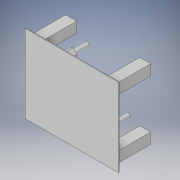
# Autodesk Inventor part: Protoboard
Saved by Autodesk Inventor 2019.3 (Build 233278000, 278)
## iProperties
Created: 2019-06-06
Part Number: Protoboard
Material: Generic
Document SubType Name: Modeling
Designer: Frienddo
Density: 1 g/cm^3
Appearance: Default
Author: Frienddo
Autodesk Inventor part; units mm, degrees
ref_plane "YZ Plane" through (0, 0, 0) normal (1, 0, 0) x (0, 1, 0)
ref_plane "XZ Plane" through (0, 0, 0) normal (0, 1, 0) x (-1, 0, 0)
ref_plane "XY Plane" through (0, 0, 0) normal (0, 0, 1) x (1, 0, 0)
sketch "Sketch1" plane through (0, 0, 0) normal (0, 0, 1) x (1, 0, 0)
  line L0 (0, 0) -> (-29.85, 0)
  line L1 (-29.85, 0) -> (-29.85, 16.75)
  line L2 (-29.85, 16.75) -> (-21.75, 16.75)
  line L3 (-21.75, 16.75) -> (-21.75, 24.5)
  line L4 (-21.75, 24.5) -> (0, 24.5)
  line L5 (0, 24.5) -> (0, 0)
  circle A0 centre (-14.35, 14.5) radius 1.5
  line L6 (0, 0) -> (29.85, 0)
  line L7 (29.85, 0) -> (29.85, 16.75)
  line L8 (29.85, 16.75) -> (21.75, 16.75)
  line L9 (21.75, 16.75) -> (21.75, 24.5)
  line L10 (21.75, 24.5) -> (0, 24.5)
  circle A1 centre (14.35, 14.5) radius 1.5
  line L11 (-29.85, 0) -> (-29.85, -16.75)
  line L12 (-29.85, -16.75) -> (-21.75, -16.75)
  line L13 (-21.75, -16.75) -> (-21.75, -24.5)
  line L14 (-21.75, -24.5) -> (0, -24.5)
  line L15 (0, -24.5) -> (0, 0)
  circle A2 centre (-14.35, -14.5) radius 1.5
  line L16 (29.85, 0) -> (29.85, -16.75)
  line L17 (29.85, -16.75) -> (21.75, -16.75)
  line L18 (21.75, -16.75) -> (21.75, -24.5)
  line L19 (21.75, -24.5) -> (0, -24.5)
  circle A3 centre (14.35, -14.5) radius 1.5
  line L20 (-21.75, -24.5) -> (-29.85, -24.5)
  line L21 (-29.85, -24.5) -> (-29.85, -16.75)
  line L22 (-29.85, -24.5) -> (-22.1, -24.5)
  line L23 (-22.1, -24.5) -> (-22.1, -17.1)
  line L24 (-22.1, -17.1) -> (-29.85, -17.1)
  line L25 (-29.85, -17.1) -> (-29.85, -24.5)
  line L26 (29.85, -16.75) -> (21.75, -16.75)
  line L27 (21.75, -16.75) -> (21.75, -24.5)
  line L28 (21.75, -24.5) -> (29.85, -24.5)
  line L29 (29.85, -24.5) -> (29.85, -16.75)
  line L30 (29.85, -24.5) -> (22.1, -24.5)
  line L31 (22.1, -24.5) -> (22.1, -17.1)
  line L32 (22.1, -17.1) -> (29.85, -17.1)
  line L33 (29.85, -17.1) -> (29.85, -24.5)
  line L34 (-29.85, 16.75) -> (-21.75, 16.75)
  line L35 (-21.75, 16.75) -> (-21.75, 24.5)
  line L36 (29.85, 16.75) -> (21.75, 16.75)
  line L37 (21.75, 16.75) -> (21.75, 24.5)
  line L38 (-21.75, 24.5) -> (-29.85, 24.5)
  line L39 (-29.85, 24.5) -> (-29.85, 16.75)
  line L40 (-29.85, 24.5) -> (-22.1, 24.5)
  line L41 (-22.1, 24.5) -> (-22.1, 17.1)
  line L42 (-22.1, 17.1) -> (-29.85, 17.1)
  line L43 (-29.85, 17.1) -> (-29.85, 24.5)
  line L44 (21.75, 16.75) -> (21.75, 24.5)
  line L45 (22.1, 24.5) -> (22.1, 17.1)
  line L46 (21.75, 24.5) -> (29.85, 24.5)
  line L47 (29.85, 16.75) -> (21.75, 16.75)
  line L48 (29.85, 24.5) -> (22.1, 24.5)
  line L49 (22.1, 17.1) -> (29.85, 17.1)
  line L50 (29.85, 24.5) -> (29.85, 16.75)
  line L51 (29.85, 17.1) -> (29.85, 24.5)
  line L52 (32.85, 27.5) -> (-32.85, 27.5)
  line L53 (-32.85, 27.5) -> (-32.85, -27.5)
  line L54 (-32.85, -27.5) -> (32.85, -27.5)
  line L55 (32.85, -27.5) -> (32.85, 27.5)
  line L56 (32.85, 27.5) -> (-32.85, -27.5) construction
  line L57 (-32.85, 27.5) -> (32.85, -27.5) construction
  dimension "d0" = 15.5
  dimension "d1" = 10
  dimension "d2" = 43.5
  dimension "d3" = 59.7
  dimension "d4" = 49
  dimension "d5" = 33.5
  dimension "d6" = 3
  dimension "d36" = 0.35
  dimension "d37" = 0.35
  dimension "d40" = 3
  dimension "d41" = 3
  constraints: 116 end point, 26 symmetric about line, 8 perpendicular, 4 centre point, 4 horizontal, 4 parallel, 2 midpoint, 3 other
  measures "d0" distance from line of L1 A0.centre
  measures "d1" distance from line of L4 A0.centre
  measures "d2" distance between parallel lines of L3 L9
  measures "d3" distance between parallel lines of L7 L1
  measures "d4" distance between parallel lines of L19 L10
  measures "d5" distance between parallel lines of L17 L8
  measures "d6" diameter of A0
  measures "d36" distance between parallel lines of L13 L23
  measures "d37" distance between parallel lines of L12 L24
  measures "d40" distance between parallel lines of L19 L54
  measures "d41" distance between parallel lines of L29 L55
sketch "Sketch6" plane through (0, 0, 0) normal (0, 0, 1) x (1, 0, 0)
  line L0 (32.85, 27.5) -> (-32.85, 27.5) projected
  line L1 (32.85, -27.5) -> (32.85, 27.5) projected
  line L2 (-32.85, -27.5) -> (32.85, -27.5) projected
  line L3 (-32.85, 27.5) -> (-32.85, -27.5) projected
  point P0 (0, 0)
extrude "Extrusion10" add sketch "Sketch6" along normal blind 0.5
sketch "Sketch7" plane through (0, 0, 0) normal (0, 0, 1) x (1, 0, 0)
  circle A0 centre (-14.35, -14.5) radius 1.5
  circle A1 centre (-14.35, -14.5) radius 2.5
  line L0 (-11.875126, -14.146447) -> (-14.703553, -16.974874)
  line L1 (-13.996447, -12.025126) -> (-16.824874, -14.853553)
  line L2 (0, 0) -> (-29.85, 0)
  dimension "d46" = 1
  dimension "d47" = 45
  constraints: 4 end point, 4 point on circle, 2 tangent, 1 centre point, 1 parallel
  measures "d46" radial gap between concentric circles of A0 A1
  measures "d47" angle of L1 L2
extrude "Extrusion11" add sketch "Sketch7" against normal blind 15 contours A0 | A0 L1 A1 L0 | A0 L0 A1 L1
sketch "Sketch8" plane through (0, 0, -15) normal (0, 0, -1) x (-1, 0, 0)
  arc A0 (13.996447, -12.025126) -> (11.875126, -14.146447) centre (14.35, -14.5) ccw
  circle A1 centre (14.35, -14.5) radius 1.25
  point P0 (0, 0)
  dimension "d50" = 2.5
  constraints: 1 centre point, 1 coincident
  measures "d50" diameter of A1
extrude "Extrusion12" add sketch "Sketch8" along normal blind 10
extrude "Extrusion13" add sketch "Sketch1" against normal blind 25 contours L24 L23 L20 L21
chamfer "Chamfer3" distance 2.9 angle 45 8 edges at (-16.1178, -16.2678, 0) (-13.2893, -15.5607, 0) (-12.5822, -12.7322, 0) (-15.4107, -13.4393, 0) (-25.975, -24.5, 0) (-22.1, -20.8, 0) (-29.85, -20.8, 0) (-25.975, -17.1, 0)
mirror "Mirror2" about plane through (0, 0, 0) normal (0, 1, 0) of "Extrusion13", "Extrusion11", "Extrusion12", "Chamfer3"
mirror "Mirror3" about plane through (0, 0, 0) normal (1, 0, 0) of "Extrusion13", "Extrusion11", "Extrusion12", "Chamfer3", "Mirror2"
body "Solid5"
